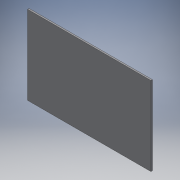
# Autodesk Inventor part: Build Plate
Saved by Autodesk Inventor 2019 (Build 230136000, 136)
## iProperties
Created: 2020-12-01
Part Number: Build Plate
Material: Generic
Document SubType Name: Modeling
Designer: Vijay
Density: 1 g/cm^3
Appearance: Default
Author: Vijay
Autodesk Inventor part; units mm, degrees
ref_plane "YZ Plane" through (0, 0, 0) normal (1, 0, 0) x (0, 1, 0)
ref_plane "XZ Plane" through (0, 0, 0) normal (0, 1, 0) x (-1, 0, 0)
ref_plane "XY Plane" through (0, 0, 0) normal (0, 0, 1) x (1, 0, 0)
sketch "Sketch1" plane through (0, 0, 0) normal (0, 0, 1) x (1, 0, 0)
  line L0 (-132.5, 80) -> (132.5, 80)
  line L1 (132.5, 80) -> (132.5, -80)
  line L2 (132.5, -80) -> (-132.5, -80)
  line L3 (-132.5, -80) -> (-132.5, 80)
  line L4 (-132.5, 80) -> (132.5, -80) construction
  line L5 (132.5, 80) -> (-132.5, -80) construction
  point P0 (0, 0)
  dimension "d0" = 265
  dimension "d1" = 160
  constraints: 12 end point, 2 midpoint, 2 parallel, 1 horizontal, 1 perpendicular
  measures "d0" distance of L0.start L0.end
  measures "d1" distance of L0.end L1.end
extrude "Extrusion1" add sketch "Sketch1" along normal blind 3
sketch "Sketch2" plane through (0, 0, 3) normal (0, 0, 1) x (1, 0, 0)
  line L0 (120, -70) -> (120, -10) construction
  line L1 (122.5, -70) -> (122.5, -10)
  line L2 (117.5, -10) -> (117.5, -70)
  arc A0 (117.5, -70) -> (122.5, -70) centre (120, -70) ccw
  arc A1 (122.5, -10) -> (117.5, -10) centre (120, -10) ccw
  line L3 (120, 10) -> (120, 70) construction
  line L4 (122.5, 10) -> (122.5, 70)
  line L5 (117.5, 70) -> (117.5, 10)
  arc A2 (117.5, 10) -> (122.5, 10) centre (120, 10) ccw
  arc A3 (122.5, 70) -> (117.5, 70) centre (120, 70) ccw
  line L6 (132.5, -80) -> (132.5, 80) projected
  line L7 (132.5, 80) -> (-132.5, 80) projected
  line L8 (-132.5, -80) -> (132.5, -80) projected
  line L9 (110, -30) -> (110, 30) construction
  line L10 (112.5, -30) -> (112.5, 30)
  line L11 (107.5, 30) -> (107.5, -30)
  arc A4 (107.5, -30) -> (112.5, -30) centre (110, -30) ccw
  arc A5 (112.5, 30) -> (107.5, 30) centre (110, 30) ccw
  arc A6 (102.5, 70) -> (97.5, 70) centre (100, 70) ccw
  arc A7 (92.5, 30) -> (87.5, 30) centre (90, 30) ccw
  line L12 (100, 10) -> (100, 70) construction
  line L13 (97.5, 70) -> (97.5, 10)
  line L14 (102.5, 10) -> (102.5, 70)
  arc A8 (102.5, -10) -> (97.5, -10) centre (100, -10) ccw
  line L15 (87.5, 30) -> (87.5, -30)
  line L16 (90, -30) -> (90, 30) construction
  line L17 (92.5, -30) -> (92.5, 30)
  arc A9 (87.5, -30) -> (92.5, -30) centre (90, -30) ccw
  line L18 (100, -70) -> (100, -10) construction
  line L19 (97.5, -10) -> (97.5, -70)
  arc A10 (97.5, -70) -> (102.5, -70) centre (100, -70) ccw
  line L20 (102.5, -70) -> (102.5, -10)
  arc A11 (97.5, 10) -> (102.5, 10) centre (100, 10) ccw
  arc A12 (82.5, 70) -> (77.5, 70) centre (80, 70) ccw
  arc A13 (72.5, 30) -> (67.5, 30) centre (70, 30) ccw
  line L21 (80, 10) -> (80, 70) construction
  line L22 (77.5, 70) -> (77.5, 10)
  line L23 (82.5, 10) -> (82.5, 70)
  arc A14 (82.5, -10) -> (77.5, -10) centre (80, -10) ccw
  line L24 (67.5, 30) -> (67.5, -30)
  line L25 (70, -30) -> (70, 30) construction
  line L26 (72.5, -30) -> (72.5, 30)
  arc A15 (67.5, -30) -> (72.5, -30) centre (70, -30) ccw
  line L27 (80, -70) -> (80, -10) construction
  line L28 (77.5, -10) -> (77.5, -70)
  arc A16 (77.5, -70) -> (82.5, -70) centre (80, -70) ccw
  line L29 (82.5, -70) -> (82.5, -10)
  arc A17 (77.5, 10) -> (82.5, 10) centre (80, 10) ccw
  arc A18 (62.5, 70) -> (57.5, 70) centre (60, 70) ccw
  arc A19 (52.5, 30) -> (47.5, 30) centre (50, 30) ccw
  line L30 (60, 10) -> (60, 70) construction
  line L31 (57.5, 70) -> (57.5, 10)
  line L32 (62.5, 10) -> (62.5, 70)
  arc A20 (62.5, -10) -> (57.5, -10) centre (60, -10) ccw
  line L33 (47.5, 30) -> (47.5, -30)
  line L34 (50, -30) -> (50, 30) construction
  line L35 (52.5, -30) -> (52.5, 30)
  arc A21 (47.5, -30) -> (52.5, -30) centre (50, -30) ccw
  line L36 (60, -70) -> (60, -10) construction
  line L37 (57.5, -10) -> (57.5, -70)
  arc A22 (57.5, -70) -> (62.5, -70) centre (60, -70) ccw
  line L38 (62.5, -70) -> (62.5, -10)
  arc A23 (57.5, 10) -> (62.5, 10) centre (60, 10) ccw
  arc A24 (42.5, 70) -> (37.5, 70) centre (40, 70) ccw
  arc A25 (32.5, 30) -> (27.5, 30) centre (30, 30) ccw
  line L39 (40, 10) -> (40, 70) construction
  line L40 (37.5, 70) -> (37.5, 10)
  line L41 (42.5, 10) -> (42.5, 70)
  arc A26 (42.5, -10) -> (37.5, -10) centre (40, -10) ccw
  line L42 (27.5, 30) -> (27.5, -30)
  line L43 (30, -30) -> (30, 30) construction
  line L44 (32.5, -30) -> (32.5, 30)
  arc A27 (27.5, -30) -> (32.5, -30) centre (30, -30) ccw
  line L45 (40, -70) -> (40, -10) construction
  line L46 (37.5, -10) -> (37.5, -70)
  arc A28 (37.5, -70) -> (42.5, -70) centre (40, -70) ccw
  line L47 (42.5, -70) -> (42.5, -10)
  arc A29 (37.5, 10) -> (42.5, 10) centre (40, 10) ccw
  arc A30 (22.5, 70) -> (17.5, 70) centre (20, 70) ccw
  arc A31 (12.5, 30) -> (7.5, 30) centre (10, 30) ccw
  line L48 (20, 10) -> (20, 70) construction
  line L49 (17.5, 70) -> (17.5, 10)
  line L50 (22.5, 10) -> (22.5, 70)
  arc A32 (22.5, -10) -> (17.5, -10) centre (20, -10) ccw
  line L51 (7.5, 30) -> (7.5, -30)
  line L52 (10, -30) -> (10, 30) construction
  line L53 (12.5, -30) -> (12.5, 30)
  arc A33 (7.5, -30) -> (12.5, -30) centre (10, -30) ccw
  line L54 (20, -70) -> (20, -10) construction
  line L55 (17.5, -10) -> (17.5, -70)
  arc A34 (17.5, -70) -> (22.5, -70) centre (20, -70) ccw
  line L56 (22.5, -70) -> (22.5, -10)
  arc A35 (17.5, 10) -> (22.5, 10) centre (20, 10) ccw
  arc A36 (2.5, 70) -> (-2.5, 70) centre (0, 70) ccw
  arc A37 (-7.5, 30) -> (-12.5, 30) centre (-10, 30) ccw
  line L57 (0, 10) -> (0, 70) construction
  line L58 (-2.5, 70) -> (-2.5, 10)
  line L59 (2.5, 10) -> (2.5, 70)
  arc A38 (2.5, -10) -> (-2.5, -10) centre (0, -10) ccw
  line L60 (-12.5, 30) -> (-12.5, -30)
  line L61 (-10, -30) -> (-10, 30) construction
  line L62 (-7.5, -30) -> (-7.5, 30)
  arc A39 (-12.5, -30) -> (-7.5, -30) centre (-10, -30) ccw
  line L63 (0, -70) -> (0, -10) construction
  line L64 (-2.5, -10) -> (-2.5, -70)
  arc A40 (-2.5, -70) -> (2.5, -70) centre (0, -70) ccw
  line L65 (2.5, -70) -> (2.5, -10)
  arc A41 (-2.5, 10) -> (2.5, 10) centre (0, 10) ccw
  arc A42 (-17.5, 70) -> (-22.5, 70) centre (-20, 70) ccw
  arc A43 (-27.5, 30) -> (-32.5, 30) centre (-30, 30) ccw
  line L66 (-20, 10) -> (-20, 70) construction
  line L67 (-22.5, 70) -> (-22.5, 10)
  line L68 (-17.5, 10) -> (-17.5, 70)
  arc A44 (-17.5, -10) -> (-22.5, -10) centre (-20, -10) ccw
  line L69 (-32.5, 30) -> (-32.5, -30)
  line L70 (-30, -30) -> (-30, 30) construction
  line L71 (-27.5, -30) -> (-27.5, 30)
  arc A45 (-32.5, -30) -> (-27.5, -30) centre (-30, -30) ccw
  line L72 (-20, -70) -> (-20, -10) construction
  line L73 (-22.5, -10) -> (-22.5, -70)
  arc A46 (-22.5, -70) -> (-17.5, -70) centre (-20, -70) ccw
  line L74 (-17.5, -70) -> (-17.5, -10)
  arc A47 (-22.5, 10) -> (-17.5, 10) centre (-20, 10) ccw
  arc A48 (-37.5, 70) -> (-42.5, 70) centre (-40, 70) ccw
  arc A49 (-47.5, 30) -> (-52.5, 30) centre (-50, 30) ccw
  line L75 (-40, 10) -> (-40, 70) construction
  line L76 (-42.5, 70) -> (-42.5, 10)
  line L77 (-37.5, 10) -> (-37.5, 70)
  arc A50 (-37.5, -10) -> (-42.5, -10) centre (-40, -10) ccw
  line L78 (-52.5, 30) -> (-52.5, -30)
  line L79 (-50, -30) -> (-50, 30) construction
  line L80 (-47.5, -30) -> (-47.5, 30)
  arc A51 (-52.5, -30) -> (-47.5, -30) centre (-50, -30) ccw
  line L81 (-40, -70) -> (-40, -10) construction
  line L82 (-42.5, -10) -> (-42.5, -70)
  arc A52 (-42.5, -70) -> (-37.5, -70) centre (-40, -70) ccw
  line L83 (-37.5, -70) -> (-37.5, -10)
  arc A53 (-42.5, 10) -> (-37.5, 10) centre (-40, 10) ccw
  arc A54 (-57.5, 70) -> (-62.5, 70) centre (-60, 70) ccw
  arc A55 (-67.5, 30) -> (-72.5, 30) centre (-70, 30) ccw
  line L84 (-60, 10) -> (-60, 70) construction
  line L85 (-62.5, 70) -> (-62.5, 10)
  line L86 (-57.5, 10) -> (-57.5, 70)
  arc A56 (-57.5, -10) -> (-62.5, -10) centre (-60, -10) ccw
  line L87 (-72.5, 30) -> (-72.5, -30)
  line L88 (-70, -30) -> (-70, 30) construction
  line L89 (-67.5, -30) -> (-67.5, 30)
  arc A57 (-72.5, -30) -> (-67.5, -30) centre (-70, -30) ccw
  line L90 (-60, -70) -> (-60, -10) construction
  line L91 (-62.5, -10) -> (-62.5, -70)
  arc A58 (-62.5, -70) -> (-57.5, -70) centre (-60, -70) ccw
  line L92 (-57.5, -70) -> (-57.5, -10)
  arc A59 (-62.5, 10) -> (-57.5, 10) centre (-60, 10) ccw
  arc A60 (-77.5, 70) -> (-82.5, 70) centre (-80, 70) ccw
  arc A61 (-87.5, 30) -> (-92.5, 30) centre (-90, 30) ccw
  line L93 (-80, 10) -> (-80, 70) construction
  line L94 (-82.5, 70) -> (-82.5, 10)
  line L95 (-77.5, 10) -> (-77.5, 70)
  arc A62 (-77.5, -10) -> (-82.5, -10) centre (-80, -10) ccw
  line L96 (-92.5, 30) -> (-92.5, -30)
  line L97 (-90, -30) -> (-90, 30) construction
  line L98 (-87.5, -30) -> (-87.5, 30)
  arc A63 (-92.5, -30) -> (-87.5, -30) centre (-90, -30) ccw
  line L99 (-80, -70) -> (-80, -10) construction
  line L100 (-82.5, -10) -> (-82.5, -70)
  arc A64 (-82.5, -70) -> (-77.5, -70) centre (-80, -70) ccw
  line L101 (-77.5, -70) -> (-77.5, -10)
  arc A65 (-82.5, 10) -> (-77.5, 10) centre (-80, 10) ccw
  arc A66 (-97.5, 70) -> (-102.5, 70) centre (-100, 70) ccw
  arc A67 (-107.5, 30) -> (-112.5, 30) centre (-110, 30) ccw
  line L102 (-100, 10) -> (-100, 70) construction
  line L103 (-102.5, 70) -> (-102.5, 10)
  line L104 (-97.5, 10) -> (-97.5, 70)
  arc A68 (-97.5, -10) -> (-102.5, -10) centre (-100, -10) ccw
  line L105 (-112.5, 30) -> (-112.5, -30)
  line L106 (-110, -30) -> (-110, 30) construction
  line L107 (-107.5, -30) -> (-107.5, 30)
  arc A69 (-112.5, -30) -> (-107.5, -30) centre (-110, -30) ccw
  line L108 (-100, -70) -> (-100, -10) construction
  line L109 (-102.5, -10) -> (-102.5, -70)
  arc A70 (-102.5, -70) -> (-97.5, -70) centre (-100, -70) ccw
  line L110 (-97.5, -70) -> (-97.5, -10)
  arc A71 (-102.5, 10) -> (-97.5, 10) centre (-100, 10) ccw
  arc A72 (-117.5, 70) -> (-122.5, 70) centre (-120, 70) ccw
  arc A73 (-127.5, 30) -> (-132.5, 30) centre (-130, 30) ccw
  line L111 (-120, 10) -> (-120, 70) construction
  line L112 (-122.5, 70) -> (-122.5, 10)
  line L113 (-117.5, 10) -> (-117.5, 70)
  arc A74 (-117.5, -10) -> (-122.5, -10) centre (-120, -10) ccw
  line L114 (-132.5, 30) -> (-132.5, -30)
  line L115 (-130, -30) -> (-130, 30) construction
  line L116 (-127.5, -30) -> (-127.5, 30)
  arc A75 (-132.5, -30) -> (-127.5, -30) centre (-130, -30) ccw
  line L117 (-120, -70) -> (-120, -10) construction
  line L118 (-122.5, -10) -> (-122.5, -70)
  arc A76 (-122.5, -70) -> (-117.5, -70) centre (-120, -70) ccw
  line L119 (-117.5, -70) -> (-117.5, -10)
  arc A77 (-122.5, 10) -> (-117.5, 10) centre (-120, 10) ccw
  point P0 (0, 0)
  point P1 (120, -40)
  point P2 (120, 40)
  point P3 (110, 0)
  point P4 (100, 40)
  point P5 (90, 0)
  point P6 (100, -40)
  point P7 (80, 40)
  point P8 (70, 0)
  point P9 (80, -40)
  point P10 (60, 40)
  point P11 (50, 0)
  point P12 (60, -40)
  point P13 (40, 40)
  point P14 (30, 0)
  point P15 (40, -40)
  point P16 (20, 40)
  point P17 (10, 0)
  point P18 (20, -40)
  point P19 (0, 40)
  point P20 (-10, 0)
  point P21 (0, -40)
  point P22 (-20, 40)
  point P23 (-30, 0)
  point P24 (-20, -40)
  point P25 (-40, 40)
  point P26 (-50, 0)
  point P27 (-40, -40)
  point P28 (-60, 40)
  point P29 (-70, 0)
  point P30 (-60, -40)
  point P31 (-80, 40)
  point P32 (-90, 0)
  point P33 (-80, -40)
  point P34 (-100, 40)
  point P35 (-110, 0)
  point P36 (-100, -40)
  point P37 (-120, 40)
  point P38 (-130, 0)
  point P39 (-120, -40)
  dimension "d4" = 5
  dimension "d5" = 5
  dimension "d6" = 10
  dimension "d7" = 10
  dimension "d8" = 10
  dimension "d9" = 20
  dimension "d10" = 60
  dimension "d11" = 5
  dimension "d12" = 5
  dimension "d13" = 60
  dimension "d14" = 50
  dimension "d17" = 20
  constraints: 312 end point, 156 point on circle, 78 centre point, 26 point on line, 12 tangent, 3 midpoint, 3 parallel, 2 vertical, 1 horizontal, 432 other
  measures "d4" diameter of A1
  measures "d5" diameter of A3
  measures "d6" distance between parallel lines of L6 L1
  measures "d7" distance from line of L7 L3.end
  measures "d8" distance from line of L8 L0.start
  measures "d9" distance of L3.start L0.end
  measures "d10" distance of L0.start L0.end
  measures "d11" diameter of A5
  measures "d12" distance between parallel lines of L2 L10
  measures "d13" distance of L11.start L11.end
  measures "d14" distance from line of L8 L9.start
  measures "d17" distance of L3.end L12.end
extrude "Extrusion2" cut sketch "Sketch2" against normal blind 3 contours A0 L2 A1 L1 | A2 L5 A3 L4 | A4 L11 A5 L10 | L14 A11 L13 A6 | L17 A9 L15 A7 | L20 A10 L19 A8 | L23 A17 L22 A12 | L26 A15 L24 A13 | L29 A16 L28 A14 | L32 A23 L31 A18 | L35 A21 L33 A19 | L38 A22 L37 A20 | L41 A29 L40 A24 | L44 A27 L42 A25 | L47 A28 L46 A26 | L50 A35 L49 A30 | L53 A33 L51 A31 | L56 A34 L55 A32 | L59 A41 L58 A36 | L62 A39 L60 A37 | L65 A40 L64 A38 | L68 A47 L67 A42 | L71 A45 L69 A43 | L74 A46 L73 A44 | L77 A53 L76 A48 | L80 A51 L78 A49 | L83 A52 L82 A50 | L86 A59 L85 A54 | L89 A57 L87 A55 | L92 A58 L91 A56 | L95 A65 L94 A60 | L98 A63 L96 A61 | L101 A64 L100 A62 | L104 A71 L103 A66 | L107 A69 L105 A67 | L110 A70 L109 A68 | L113 A77 L112 A72 | L119 A76 L118 A74
fillet "Fillet1" radius 5 2 edges at (-132.5, 80, 1.5) (132.5, 80, 1.5)
sketch "Sketch3" plane through (0, 0, 3) normal (0, 0, 1) x (1, 0, 0)
  line L0 (-132.5, -80) -> (132.5, -80) projected
  line L1 (132.5, -80) -> (-132.5, -80)
  line L2 (-132.5, -80) -> (-132.5, -110)
  line L3 (-132.5, -110) -> (132.5, -110)
  line L4 (132.5, -110) -> (132.5, -80)
  point P0 (0, 0)
  dimension "d25" = 30
  constraints: 8 end point, 2 parallel, 1 horizontal, 1 perpendicular
  measures "d25" distance of L3.end L0.end
extrude "Extrusion3" add sketch "Sketch3" against normal blind 3
body "Solid1"
